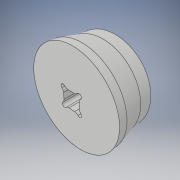
# Autodesk Inventor part: Power_Button
Saved by Autodesk Inventor 2019 (Build 230136000, 136)
## iProperties
Created: 2025-01-19
Part Number: Power_Button
Material: Générique
Document SubType Name: Modeling
Designer: Maxime
Density: 1 g/cm^3
Appearance: Par défaut
Author: Maxime
## iProperties of the stored document Power_Button_Impression 3D.ipt
Created: 2025-03-03
Part Number: Power_Button_Impression 3D
Material: Générique
Document SubType Name: Modeling
Designer: Maxime
Density: 1 g/cm^3
Appearance: Par défaut
Author: Maxime
Autodesk Inventor part; units mm, degrees
ref_plane "YZ Plane" through (0, 0, 0) normal (1, 0, 0) x (0, 1, 0)
ref_plane "XZ Plane" through (0, 0, 0) normal (0, 1, 0) x (-1, 0, 0)
ref_plane "XY Plane" through (0, 0, 0) normal (0, 0, 1) x (1, 0, 0)
sketch "Esquisse1" plane through (0, 0, 0) normal (0, 0, 1) x (1, 0, 0)
  circle A0 centre (0, 0) radius 8.85
  dimension "d0" = 17.7
  constraints: 1 centre point, 1 coincident
  measures "d0" diameter of A0
extrude "Extrusion1" add sketch "Esquisse1" along normal blind 7.05 draft 10
sketch "Esquisse2" plane through (0, 0, 7.05) normal (0, 0, 1) x (1, 0, 0)
  line L0 (1.775, -1.775) -> (-1.775, -1.775)
  line L1 (-1.775, -1.775) -> (-1.775, 1.775)
  line L2 (-1.775, 1.775) -> (1.775, 1.775)
  line L3 (1.775, 1.775) -> (1.775, -1.775)
  line L4 (1.775, -1.775) -> (-1.775, 1.775) construction
  line L5 (-1.775, -1.775) -> (1.775, 1.775) construction
  point P0 (0, 0)
  dimension "d3" = 3.55
  dimension "d4" = 3.55
  constraints: 12 end point, 2 midpoint, 2 parallel, 1 horizontal, 1 perpendicular
  measures "d3" distance of L1.end L2.end
  measures "d4" distance of L0.end L1.end
extrude "Extrusion2" cut sketch "Esquisse2" against normal blind 5.5
ref_plane "Plan de construction1" through (0, 0, 4) normal (0, 0, -1) x (-1, 0, 0)
sketch "Esquisse3" plane through (0, 0, 4) normal (0, 0, -1) x (-1, 0, 0)
  circle A0 centre (0, 0) radius 9.5553 projected
  circle A1 centre (0, 0) radius 13.8909
  line L0 (-1.775, 1.775) -> (-1.775, -1.775) projected
  line L1 (-1.775, -1.775) -> (1.775, -1.775) projected
  line L2 (1.775, -1.775) -> (1.775, 1.775) projected
  line L3 (1.775, 1.775) -> (-1.775, 1.775) projected
  constraints: 1 centre point, 1 coincident
extrude "Extrusion3" cut sketch "Esquisse3" against normal through all contours A1
sketch "Esquisse4" plane through (0, 0, 0) normal (0, 0, -1) x (-1, 0, 0)
  circle A0 centre (0, 0) radius 8.85 projected
extrude "Extrusion4" add sketch "Esquisse4" along normal blind 2.5
sketch "Esquisse5" plane through (0, 0, -2.5) normal (0, 0, -1) x (-1, 0, 0)
  line L0 (2.6892, 4.9729) -> (2.6892, -4.9729) construction
  line L1 (2.6892, -4.9729) -> (-2.6892, -4.9729) construction
  line L2 (-2.6892, -4.9729) -> (-2.6892, 4.9729) construction
  line L3 (-2.6892, 4.9729) -> (2.6892, 4.9729) construction
  line L4 (13.3774, 0) -> (-13.3774, 0) projected
  line L5 (0, -13.3774) -> (0, 13.3774) projected
  point P0 (0, 0)
  point P1 (-3.9441, 0)
  point P2 (0, -4.9729)
  point P3 (-2.6892, 0)
  point P4 (0, -4.9729)
  constraints: 4 point on line, 2 midpoint, 2 other
extrude "Extrusion5" [suppressed]
sketch "Esquisse6" plane through (0, 0, 7.05) normal (0, 0, 1) x (1, 0, 0)
  line L0 (-1.775, 1.775) -> (1.775, 1.775) projected
  line L1 (1.775, -1.775) -> (-1.775, -1.775) projected
  point P0 (0, 0)
  constraints: 2 coincident
hole "Perçage1" at (-1.775, 1.775, 7.05) at (1.775, 1.775, 7.05) at (-1.775, -1.775, 7.05) at (1.775, -1.775, 7.05) direction (0, 0, -1) diameter 1 depth 5.5 start extended yes
fillet "Congé1" radius 1 8 edges at (-1.275, 1.775, 4.3) (1.275, 1.775, 4.3) (1.775, 1.275, 4.3) (1.775, -1.275, 4.3) (1.275, -1.775, 4.3) (-1.275, -1.775, 4.3) (-1.775, -1.275, 4.3) (-1.775, 1.275, 4.3)
sketch "Esquisse8" plane through (0, 0, 7.05) normal (0, 0, 1) x (1, 0, 0)
  circle A0 centre (0, 0) radius 10
  dimension "d29" = 20
  constraints: 1 centre point, 1 coincident
  measures "d29" diameter of A0
extrude "Extrusion7" cut sketch "Esquisse8" against normal blind 1.5
sketch "Esquisse7" plane through (0, 0, 7.05) normal (0, 0, 1) x (1, 0, 0)
  arc A0 (3.0373, 1.3601) -> (3.0546, -1.3184) centre (5.8249, 0.0388) ccw construction
  arc A1 (2.6759, 1.5314) -> (2.6954, -1.4944) centre (5.8249, 0.0388) ccw
  arc A2 (3.3988, 1.1887) -> (3.4138, -1.1424) centre (5.8249, 0.0388) ccw
  arc A3 (3.3988, 1.1887) -> (2.6759, 1.5314) centre (3.0373, 1.3601) ccw
  arc A4 (2.6954, -1.4944) -> (3.4138, -1.1424) centre (3.0546, -1.3184) ccw
  point P0 (0, 0)
  dimension "d23" = 0.8
  constraints: 10 point on circle, 5 centre point, 4 tangent
  measures "d23" diameter of A4
equation "\"d3\" = d4"
